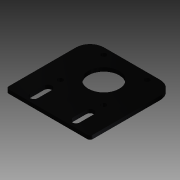
# Autodesk Inventor part: nema17_y_axis_motor_mount_12ga
Saved by Autodesk Inventor 2014 (Build 180170000, 170)
## iProperties
Created: 2013-07-14
Part Number: nema17_y_axis_motor_mount_12ga
Material: UHMW, Black
Document SubType Name: Modeling
Designer: Edward
Density: 0.94 g/cm^3
Appearance: Smooth - Black
Author: Edward
Autodesk Inventor part; units mm, degrees
ref_plane "YZ Plane" through (0, 0, 0) normal (1, 0, 0) x (0, 1, 0)
ref_plane "XZ Plane" through (0, 0, 0) normal (0, 1, 0) x (-1, 0, 0)
ref_plane "XY Plane" through (0, 0, 0) normal (0, 0, 1) x (1, 0, 0)
sketch "Sketch1" plane through (0, 0, 0) normal (0, 0, 1) x (1, 0, 0)
  line L0 (-30, 30) -> (30, 30)
  line L1 (30, 30) -> (30, -30)
  line L2 (30, -30) -> (-30, -30)
  line L3 (-30, -30) -> (-30, 30)
  point P0 (0, 0)
  dimension "d0" = 60
  dimension "d1" = 60
  dimension "d2" = 30
  dimension "d3" = 30
  constraints: 8 end point, 2 parallel, 1 horizontal, 1 perpendicular
  measures "d0" distance of L1.end L2.end
  measures "d1" distance of L0.end L1.end
  measures "d2" distance from line of point (0, 0) L3
  measures "d3" distance from line of L0 point (0, 0)
extrude "Extrusion1" add sketch "Sketch1" along normal blind 2.6568
fillet "Fillet1" radius 2 2 edges at (30, -30, 1.3284) (-30, -30, 1.3284)
sketch "Sketch3" plane through (0, 0, 2.6568) normal (0, 0, 1) x (1, 0, 0)
  line L0 (-28, -30) -> (28, -30) projected
  line L1 (30, -28) -> (30, 30) projected
  line L2 (-30, 30) -> (-30, -28) projected
  line L3 (-15, -15) -> (-15, -25) construction
  line L4 (-17.75, -15) -> (-17.75, -25)
  line L5 (-12.25, -25) -> (-12.25, -15)
  arc A0 (-12.25, -15) -> (-17.75, -15) centre (-15, -15) ccw
  arc A1 (-17.75, -25) -> (-12.25, -25) centre (-15, -25) ccw
  line L6 (15, -15) -> (15, -25) construction
  line L7 (12.25, -15) -> (12.25, -25)
  line L8 (17.75, -25) -> (17.75, -15)
  arc A2 (17.75, -15) -> (12.25, -15) centre (15, -15) ccw
  arc A3 (12.25, -25) -> (17.75, -25) centre (15, -25) ccw
  point P0 (0, 0)
  point P1 (-15, -20)
  point P2 (15, -20)
  dimension "d14" = 10
  dimension "d15" = 5.5
  dimension "d16" = 5
  dimension "d17" = 15
  dimension "d18" = 5.5
  dimension "d19" = 45
  dimension "d20" = 10
  dimension "d21" = 5
  constraints: 16 end point, 8 point on circle, 8 tangent, 4 centre point, 4 parallel, 2 midpoint
  measures "d14" distance of L3.start L3.end
  measures "d15" diameter of A1
  measures "d16" distance from line of L0 L3.end
  measures "d17" distance from line of L2 L3.end
  measures "d18" diameter of A3
  measures "d19" distance from line of L2 L6.end
  measures "d20" distance of L6.start L6.end
  measures "d21" distance from line of L0 L6.end
extrude "Extrusion3" cut sketch "Sketch3" against normal through all
sketch "Sketch4" plane through (0, 0, 2.6568) normal (0, 0, 1) x (1, 0, 0)
  line L0 (30, -28) -> (30, 30) projected
  circle A0 centre (0, 9.85) radius 11
  line L1 (-28, -30) -> (28, -30) projected
  point P0 (0, 0)
  dimension "d24" = 22
  dimension "d25" = 30
  dimension "d31" = 39.85
  constraints: 1 centre point
  measures "d24" diameter of A0
  measures "d25" distance from line of L0 A0.centre
  measures "d31" distance from line of L1 A0.centre
extrude "Extrusion4" cut sketch "Sketch4" against normal blind 7
sketch "Sketch6" plane through (0, 0, 2.6568) normal (0, 0, 1) x (1, 0, 0)
  circle A0 centre (-15.5, -5.65) radius 1.75
  circle A1 centre (0, 9.85) radius 11 projected
  point P0 (0, 0)
  dimension "d32" = 3.5
  dimension "d44" = 15.5
  dimension "d45" = 15.5
  constraints: 1 centre point
  measures "d32" diameter of A0
  measures "d44" horizontal distance of A1.centre A0.centre
  measures "d45" horizontal distance of A0.centre A1.centre
extrude "Extrusion6" cut sketch "Sketch6" against normal through all contours A0
pattern_linear "Rectangular Pattern1" count 2 spacing 31 along (1, 0, 0) count 2 spacing 31 along (0, 1, 0) of "Extrusion6"
fillet "Fillet2" radius 10 2 edges at (30, 30, 1.3284) (-30, 30, 1.3284)
equation "\"d2\" = 0.5 * d0"
equation "\"d3\" = 0.5 * d1"
body "Solid1"
